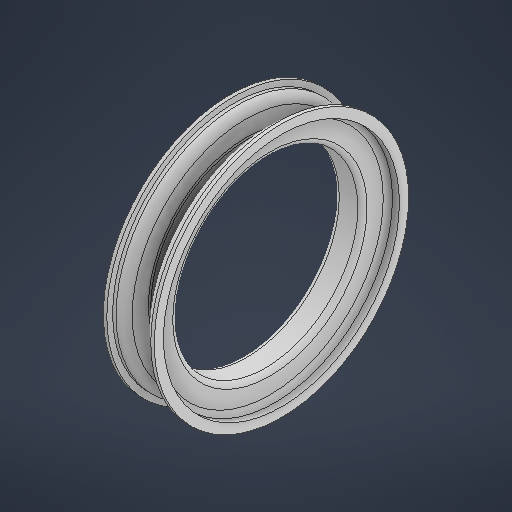
# Autodesk Inventor part: p_stratorCase
Saved by Autodesk Inventor 2026 (Build 300175000, 175)
## iProperties
Created: 2025-05-06
Part Number: p_stratorCase
Material: Generisch
Document SubType Name: Modeling
Designer: FAL
Density: 1 g/cm^3
Appearance: Vorgabe
Author: FAL
Autodesk Inventor part; units mm, degrees
ref_plane "YZ Plane" through (0, 0, 0) normal (1, 0, 0) x (0, 1, 0)
ref_plane "XZ Plane" through (0, 0, 0) normal (0, 1, 0) x (-1, 0, 0)
ref_plane "XY Plane" through (0, 0, 0) normal (0, 0, 1) x (1, 0, 0)
sketch "Skizze1" plane through (0, 0, 0) normal (0, 0, 1) x (1, 0, 0)
  line L0 (0, 0) -> (-28.0736, 0) construction
  line L1 (-11, 55) -> (0, 55)
  line L2 (0, 55) -> (0, 40)
  line L3 (0, 40) -> (-6, 40)
  line L4 (-6, 40) -> (-6, 51)
  line L5 (-6, 51) -> (-11, 51)
  line L6 (-11, 51) -> (-11, 55)
  line L7 (0, 40) -> (0, 0) construction
  dimension "d4" = 4
  dimension "d5" = 5
  dimension "d6" = 6
  dimension "d7" = 15
  dimension "d8" = 80
  constraints: 16 end point, 5 perpendicular, 2 horizontal, 1 vertical
  measures "d4" distance between parallel lines of L1 L5
  measures "d5" distance between parallel lines of L4 L6
  measures "d6" distance between parallel lines of L2 L4
  measures "d7" distance between parallel lines of L3 L1
  measures "d8" diameter of L3 L0
revolve "Umdrehung1" add sketch "Skizze1" angle 360 about axis through (0, 0, 0) along (-1, 0, 0)
fillet "Rundung2" radius 2 1 edges at (-6, -51, 0)
fillet "Rundung3" radius 2 1 edges at (-6, -40, 0)
shell "Wandung2" thickness 1.5 removed faces 2 at (0, -49.7558, 1.4416) at (-3.6667, -50.386, 22.0512)
mirror "Spiegeln1" about plane through (0, 55, 0) normal (1, 0, 0)
